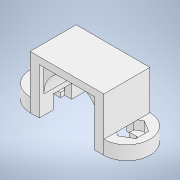
# Autodesk Inventor part: Кронштейн для двигателей серии N
Saved by Autodesk Inventor 2020 (Build 240168000, 168)
## iProperties
Created: 2019-11-25
Part Number: Кронштейн для двигателей серии N
Material: Типовые
Document SubType Name: Modeling
Designer: ivanc
Density: 1 g/cm^3
Appearance: Белый
Author: ivanc
Autodesk Inventor part; units mm, degrees
ref_plane "YZ Plane" through (0, 0, 0) normal (1, 0, 0) x (0, 1, 0)
ref_plane "XZ Plane" through (0, 0, 0) normal (0, 1, 0) x (-1, 0, 0)
ref_plane "XY Plane" through (0, 0, 0) normal (0, 0, 1) x (1, 0, 0)
sketch "Эскиз1" plane through (0, 0, 0) normal (0, 0, 1) x (1, 0, 0)
  circle A0 centre (0, 0) radius 6
  line L0 (-6, 0) -> (6, 0)
  line L1 (6, 0) -> (6, 5)
  line L2 (6, 5) -> (-6, 5)
  line L3 (-6, 5) -> (-6, 0)
  line L4 (-6, 0) -> (6, 0)
  line L5 (6, 0) -> (6, -4)
  line L6 (6, -4) -> (-6, -4)
  line L7 (-6, -4) -> (-6, 0)
  line L8 (-6, -4) -> (-8, -4)
  line L9 (-8, -4) -> (-8, 5)
  line L10 (-8, 5) -> (-6, 5)
  line L11 (-6, 5) -> (-6, -4)
  line L12 (6, 5) -> (8, 5)
  line L13 (8, 5) -> (8, -4)
  line L14 (8, -4) -> (6, -4)
  line L15 (6, -4) -> (6, 5)
  line L16 (-8, 5) -> (8, 5)
  line L17 (8, 5) -> (8, 7.5)
  line L18 (8, 7.5) -> (-8, 7.5)
  line L19 (-8, 7.5) -> (-8, 5)
  line L20 (-8, -4) -> (-13, -4)
  line L21 (-13, -4) -> (-13, -1)
  line L22 (-13, -1) -> (-8, -1)
  line L23 (-8, -1) -> (-8, -4)
  line L24 (8, -4) -> (13, -4)
  line L25 (13, -4) -> (13, -1)
  line L26 (13, -1) -> (8, -1)
  line L27 (8, -1) -> (8, -4)
  point P0 (8, -1)
  point P1 (-8, -1)
  point P2 (-3.3166, 5)
  point P3 (3.3166, 5)
  dimension "d0" = 12
  dimension "d1" = 5
  dimension "d2" = 4
  dimension "d3" = 2
  dimension "d4" = 2
  dimension "d5" = 2.5
  dimension "d8" = 5
  dimension "d9" = 5
  dimension "d37" = 3
  constraints: 56 end point, 14 parallel, 7 horizontal, 7 perpendicular, 3 collinear, 2 coincident, 2 point on line, 1 midpoint, 3 other
  measures "d1" distance of L1.end L0.end
  measures "d2" distance of L4.end L5.end
  measures "d3" distance of L9.end L10.end
  measures "d4" distance of L13.end L14.end
  measures "d5" distance of L17.end L16.end
  measures "d8" distance of L21.end L22.end
  measures "d9" distance of L26.end L25.end
  measures "d37" distance between parallel lines of L24 L26
extrude "Выдавливание1" add sketch "Эскиз1" along normal blind 10 contours A0 L2 L1 | L1 L12 L13 L14 L5 | L2 A0 | A0 L2 L10 L19 L18 L17 L12 | L3 L2 A0 | L7 L8 L9 L10 L3 | L13 L26 L25 L24 | L20 L21 L22 L9
sketch "Эскиз2" plane through (-13, -1, 0) normal (0, 1, 0) x (1, 0, 0)
  line L0 (5, 0) -> (0, 0) projected
  line L1 (2.5, 0) -> (2.5, -10)
  line L2 (5, -10) -> (0, -10) projected
  line L3 (26, -10) -> (21, -10) projected
  line L4 (23.5, -10) -> (23.5, 0)
  line L5 (26, 0) -> (21, 0) projected
  line L6 (23.5, -5) -> (21.9, -5)
  line L7 (2.5, -5) -> (4.1, -5)
  point P0 (13, 0)
  dimension "d17" = 1.6
  dimension "d18" = 1.6
  constraints: 8 end point, 6 midpoint, 2 coincident, 2 horizontal
  measures "d17" distance of L6.start L6.end
  measures "d18" distance of L7.start L7.end
hole "Отверстие2" at (-8.9, -1, 5) at (8.9, -1, 5) direction (0, -1, 0) diameter 2.2 end through all
sketch "Эскиз3" plane through (8, -1, 0) normal (0, 1, 0) x (1, 0, 0)
  arc A0 (-16, -4.3675) -> (-16, -5.6325) centre (-16.9, -5) ccw projected
  arc A1 (0, -5.6325) -> (0, -4.3675) centre (0.9, -5) ccw projected
  line L0 (3.35, -6.4145) -> (0.9, -7.829)
  line L1 (0.9, -7.829) -> (-1.55, -6.4145)
  line L2 (-1.55, -6.4145) -> (-1.55, -3.5855)
  line L3 (-1.55, -3.5855) -> (0.9, -2.171)
  line L4 (0.9, -2.171) -> (3.35, -3.5855)
  line L5 (3.35, -3.5855) -> (3.35, -6.4145)
  line L6 (-19.35, -3.5855) -> (-16.9, -2.171)
  line L7 (-16.9, -2.171) -> (-14.45, -3.5855)
  line L8 (-14.45, -3.5855) -> (-14.45, -6.4145)
  line L9 (-14.45, -6.4145) -> (-16.9, -7.829)
  line L10 (-16.9, -7.829) -> (-19.35, -6.4145)
  line L11 (-19.35, -6.4145) -> (-19.35, -3.5855)
  line L12 (-21, 0) -> (-21, -10) projected
  line L13 (5, 0) -> (5, -10) projected
  point P0 (-8, 0)
  dimension "d26" = 4.9
  constraints: 24 end point, 3 parallel, 2 coincident, 26 other
  measures "d26" distance between parallel lines of L2 L5
extrude "Выдавливание2" cut sketch "Эскиз3" against normal blind 2
fillet "Сопряжение1" radius 5 4 edges at (-13, -2.5, 0) (-13, -2.5, 10) (13, -2.5, 0) (13, -2.5, 10)
sketch "Эскиз5" plane through (0, 0, 10) normal (0, 0, 1) x (1, 0, 0)
  line L0 (-6, -4) -> (-6, 0) projected
  line L1 (-6, 0) -> (6, 0)
  line L2 (6, 0) -> (6, 6)
  line L3 (6, 6) -> (-6, 6)
  line L4 (-6, 6) -> (-6, 0)
  line L5 (6, 0) -> (6, -4) projected
  line L6 (-3.3166, 5) -> (3.3166, 5) projected
  point P0 (0, 0)
  dimension "d34" = 1
  constraints: 8 end point, 2 parallel, 1 collinear, 1 horizontal, 1 perpendicular
  measures "d34" distance between parallel lines of L6 L3
extrude "Выдавливание4" cut sketch "Эскиз5" against normal blind 1
sketch "Эскиз6" plane through (-6, -4, 0) normal (0, -1, 0) x (1, 0, 0)
  line L0 (-1.5, 7) -> (0, 7)
  line L1 (0, 7) -> (0, 3)
  line L2 (0, 3) -> (-1.5, 3)
  line L3 (-1.5, 3) -> (-1.5, 7)
  line L4 (0, 0) -> (0, 10) projected
  line L5 (-2.9, 3.9) -> (-1.5, 3.9)
  line L6 (-1.5, 3.9) -> (-1.5, 6.1)
  line L7 (-1.5, 6.1) -> (-2.9, 6.1)
  line L8 (-2.9, 6.1) -> (-2.9, 3.9)
  circle A0 centre (-2.9, 5) radius 1.1 projected
  line L9 (14, 0) -> (-2, 0) projected
  line L10 (6, 0) -> (6, 10)
  line L11 (0, 10) -> (12, 10) projected
  line L12 (13.5, 7) -> (12, 7)
  line L13 (12, 7) -> (12, 3)
  line L14 (12, 3) -> (13.5, 3)
  line L15 (13.5, 3) -> (13.5, 7)
  line L16 (14.9, 3.9) -> (13.5, 3.9)
  line L17 (13.5, 3.9) -> (13.5, 6.1)
  line L18 (13.5, 6.1) -> (14.9, 6.1)
  line L19 (14.9, 6.1) -> (14.9, 3.9)
  point P0 (0, 5)
  point P1 (-2.9, 3.9)
  point P2 (-2.9, 6.1)
  point P3 (-2.9, 3.9)
  point P4 (-2.9, 6.1)
  point P5 (12, 5)
  point P6 (14.9, 5)
  point P7 (14.9, 5)
  dimension "d38" = 4
  dimension "d42" = 1.5
  constraints: 34 end point, 11 symmetric about line, 5 midpoint, 4 parallel, 2 coincident, 2 horizontal, 2 perpendicular, 1 collinear, 1 tangent
  measures "d38" distance of L0.end L1.end
  measures "d42" distance of L1.end L2.end
extrude "Выдавливание5" cut sketch "Эскиз6" against normal up to surface (3 mm away) contours L0 L1 L2 L3 | L3 L5 A0 L7 | A0 L8 | L15 L14 L13 L12 | L18 L19 L16 L15 picked at (-2.5898, 5.2959)
